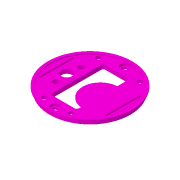
# Autodesk Inventor part: top_ring
Saved by Autodesk Inventor 2018 (Build 220112000, 112)
## iProperties
Created: 2019-01-25
Part Number: top_ring
Material: Generic
Document SubType Name: Modeling
Designer: Koki
Density: 1 g/cm^3
Appearance: Magenta
Author: Koki
Autodesk Inventor part; units mm, degrees
ref_plane "YZ Plane" through (0, 0, 0) normal (1, 0, 0) x (0, 1, 0)
ref_plane "XZ Plane" through (0, 0, 0) normal (0, 1, 0) x (-1, 0, 0)
ref_plane "XY Plane" through (0, 0, 0) normal (0, 0, 1) x (1, 0, 0)
ref_plane "Work Plane5" through (0, 4, 0) normal (0, 1, 0) x (1, 0, 0)
sketch "Sketch6" plane through (0, 4, 0) normal (0, 1, 0) x (1, 0, 0)
  circle A0 centre (0, 0) radius 38.1
  line L0 (15.875, -27.4963) -> (17.4625, -30.2459)
  line L1 (-15.875, -27.4963) -> (-17.4625, -30.2459)
  arc A1 (15.875, -27.4963) -> (27.4963, 15.875) centre (0, 0) ccw
  arc A2 (-27.4963, 15.875) -> (-15.875, -27.4963) centre (0, 0) ccw
  arc A3 (17.4625, -30.2459) -> (30.2459, 17.4625) centre (0, 0) ccw
  arc A4 (-30.2459, 17.4625) -> (-17.4625, -30.2459) centre (0, 0) ccw
  line L2 (0, 0) -> (-30.2459, 17.4625)
  line L3 (0, 0) -> (30.2459, 17.4625)
  line L4 (-15.875, 0) -> (19.5597, 0)
  dimension "d89" = 30
  dimension "d90" = 30
  constraints: 10 end point, 8 point on circle, 5 centre point, 3 coincident, 2 point on line, 1 horizontal
  measures "d89" angle of L4 L2
  measures "d90" angle of L4 L3
extrude "Extrusion6" add sketch "Sketch6" against normal blind 4 contours A0 | A1 L3 A3 L0 | L1 A4 L2 A2
sketch "Sketch7" plane through (0, 0, 0) normal (0, 0, 1) x (1, 0, 0)
  line L0 (0, 0) -> (0, 4)
  line L1 (-38.1, 4) -> (38.1, 4) projected
  line L2 (38.1, 4) -> (37.1, 4)
  line L3 (37.1, 4) -> (37.1, 5)
  line L4 (37.1, 5) -> (38.1, 5)
  line L5 (38.1, 5) -> (38.1, 4)
  line L6 (38.1, 4) -> (39.6875, 4)
  line L7 (39.6875, 4) -> (39.6875, 5)
  line L8 (39.6875, 5) -> (38.1, 5)
  line L9 (38.1, 5) -> (38.1, 4)
  dimension "d43" = 1
  dimension "d44" = 1
  dimension "d45" = 1.5875
  constraints: 18 end point, 4 parallel, 2 horizontal, 2 perpendicular, 1 point on line
  measures "d43" distance of L2.end L3.end
  measures "d44" distance of L3.end L4.end
  measures "d45" distance of L7.end L8.end
revolve "Revolution1" add sketch "Sketch7" angle 360 about axis through (0, 0, 0) along (0, 1, 0)
ref_plane "Work Plane3" through (0, 4, 0) normal (0, 1, 0) x (1, 0, 0)
sketch "Sketch10" plane through (0, 4, 0) normal (0, 1, 0) x (1, 0, 0)
  circle A0 centre (12.7, -30.48) radius 2.2
  line L0 (0, 0) -> (19.9404, 0)
  line L1 (0, 0) -> (0, -20.9357)
  circle A1 centre (12.7, 30.48) radius 2.2
  circle A2 centre (-12.7, -30.48) radius 2.2
  circle A3 centre (-12.7, 30.48) radius 2.2
  dimension "d46" = 30.48
  dimension "d47" = 12.7
  dimension "d48" = 4.4
  constraints: 4 centre point, 4 end point, 3 symmetric about line, 1 horizontal, 1 vertical, 3 other
  measures "d46" vertical distance of L0.start A0.centre
  measures "d47" horizontal distance of L0.start A0.centre
  measures "d48" diameter of A0
extrude "Extrusion7" cut sketch "Sketch10" against normal blind 4 contours A0 | A2
sketch "Sketch13" plane through (0, 4, 0) normal (0, 1, 0) x (1, 0, 0)
  line L0 (-32.258, -16.51) -> (-30.48, -16.51)
  line L1 (-30.48, -16.51) -> (-30.48, 16.51)
  line L2 (-30.48, 16.51) -> (-32.258, 16.51)
  line L3 (-32.258, 16.51) -> (-32.258, -16.51)
  point P0 (0, 0)
  dimension "d58" = 1.778
  dimension "d59" = 33.02
  dimension "d60" = 16.51
  dimension "d61" = 30.48
  constraints: 8 end point, 2 parallel, 1 horizontal, 1 perpendicular
  measures "d58" distance between parallel lines of L1 L3
  measures "d59" distance of L2.end L0.start
  measures "d60" distance from line of point (0, 0) L0
  measures "d61" distance from line of point (0, 0) L1
extrude "Extrusion10" cut sketch "Sketch13" along normal mid plane 3
mirror "Mirror1" about plane through (0, 0, 0) normal (1, 0, 0) of "Extrusion10"
chamfer "Chamfer2" distance 0.5 angle 45 4 edges at (-32.258, 4, 0) (-30.48, 4, 0) (32.258, 4, 0) (30.48, 4, 0)
sketch "Sketch14" plane through (0, 0, 0) normal (0, -1, 0) x (1, 0, 0)
  circle A0 centre (0, 33.02) radius 2.425
  point P0 (0, 0)
  dimension "d70" = 4.85
  dimension "d71" = 33.02
  constraints: 1 centre point
  measures "d70" diameter of A0
  measures "d71" distance of point (0, 0) A0.centre
extrude "Extrusion11" cut sketch "Sketch14" against normal blind 25.75
pattern_circular "Circular Pattern4" count 2 over 360 about axis through (0, 4.5, 0) along (0, -1, 0) of "Extrusion11"
sketch "Sketch15" plane through (0, 0, 0) normal (0, -1, 0) x (1, 0, 0)
  circle A0 centre (-12.7, 30.48) radius 2.2 projected
  circle A1 centre (-12.7, 30.48) radius 4
  line L0 (0, 0) -> (0, 13.7604)
  line L1 (0, 0) -> (23.7395, 0)
  circle A2 centre (12.7, 30.48) radius 4
  circle A3 centre (-12.7, -30.48) radius 2.2
  circle A4 centre (-12.7, -30.48) radius 4
  circle A5 centre (12.7, -30.48) radius 4
  dimension "d77" = 8
  constraints: 5 centre point, 4 end point, 4 symmetric about line, 2 coincident, 1 horizontal, 1 vertical, 4 other
  measures "d77" diameter of A1
extrude "Extrusion12" cut sketch "Sketch15" against normal blind 3 contours A1 | A2
sketch "Sketch16" plane through (0, 4, 0) normal (0, 1, 0) x (1, 0, 0)
  circle A0 centre (0, 33.02) radius 2.425 projected
  line L0 (0, 28.6899) -> (-3.75, 30.8549)
  line L1 (-3.75, 30.8549) -> (-3.75, 35.1851)
  line L2 (-3.75, 35.1851) -> (0, 37.3501)
  line L3 (0, 37.3501) -> (3.75, 35.1851)
  line L4 (3.75, 35.1851) -> (3.75, 30.8549)
  line L5 (3.75, 30.8549) -> (0, 28.6899)
  line L6 (0, 0) -> (11.6751, 0)
  circle A1 centre (0, -33.02) radius 2.425
  line L7 (0, -28.6899) -> (-3.75, -30.8549)
  line L8 (-3.75, -30.8549) -> (-3.75, -35.1851)
  line L9 (-3.75, -35.1851) -> (0, -37.3501)
  line L10 (0, -37.3501) -> (3.75, -35.1851)
  line L11 (3.75, -35.1851) -> (3.75, -30.8549)
  line L12 (3.75, -30.8549) -> (0, -28.6899)
  dimension "d80" = 7.5
  constraints: 26 end point, 8 symmetric about line, 2 coincident, 1 centre point, 1 horizontal, 14 other
  measures "d80" distance between parallel lines of L4 L1
extrude "Extrusion13" cut sketch "Sketch16" against normal blind 2.2
sketch "Sketch18" plane through (0, 4, 0) normal (0, 1, 0) x (1, 0, 0)
  circle A0 centre (19.558, 27.6098) radius 2.2
  line L0 (0, 0) -> (19.3787, 0)
  line L1 (0, 0) -> (0, 25.4098)
  circle A1 centre (-19.558, 27.6098) radius 2.2
  dimension "d83" = 4.4
  dimension "d84" = 27.6098
  dimension "d85" = 19.558
  constraints: 4 end point, 2 centre point, 1 horizontal, 1 symmetric about line, 1 vertical, 1 other
  measures "d83" diameter of A0
  measures "d84" vertical distance of L0.start A0.centre
  measures "d85" horizontal distance of L0.start A0.centre
extrude "Extrusion14" cut sketch "Sketch18" against normal blind 10
sketch "Sketch20" plane through (0, 0, 0) normal (0, 1, 0) x (-1, 0, 0)
  line L0 (12.5, 25) -> (-12.5, 25)
  line L1 (-12.5, 25) -> (-12.5, -25)
  line L2 (-12.5, -25) -> (12.5, -25)
  line L3 (12.5, -25) -> (12.5, 25)
  point P0 (0, 0)
  dimension "d94" = 50
  dimension "d95" = 25
  dimension "d96" = 25
  dimension "d97" = 12.5
  constraints: 8 end point, 2 parallel, 1 horizontal, 1 perpendicular
  measures "d94" distance of L0.end L1.end
  measures "d95" distance of L0.start L0.end
  measures "d96" distance from line of point (0, 0) L0
  measures "d97" distance from line of point (0, 0) L1
extrude "Extrusion15" cut sketch "Sketch20" along normal blind 10
fillet "Fillet5" radius 2 4 edges at (12.5, 2, 25) (-12.5, 2, 25) (-12.5, 2, -25) (12.5, 2, -25)
sketch "Sketch21" plane through (0, 0, 0) normal (0, -1, 0) x (1, 0, 0)
  circle A0 centre (-19.558, -27.6098) radius 2.2 projected
  circle A1 centre (-19.558, -27.6098) radius 4
  circle A2 centre (19.558, -27.6098) radius 2.2 projected
  circle A3 centre (19.558, -27.6098) radius 4
  circle A4 centre (-12.7, 30.48) radius 4 projected
  point P0 (0, 0)
  dimension "d102" = 8
  dimension "d103" = 8
  constraints: 2 centre point, 2 coincident
  measures "d102" diameter of A1
  measures "d103" diameter of A3
extrude "Extrusion16" cut sketch "Sketch21" against normal blind 3 contours A1 | A3
sketch "Sketch22" plane through (0, 4, 0) normal (0, 1, 0) x (1, 0, 0)
  circle A0 centre (22, 0) radius 5
  line L0 (0, 0) -> (0, -19.8965)
  circle A1 centre (-22, 0) radius 5
  circle A2 centre (20, 12) radius 2.75
  line L1 (0, 0) -> (8.5328, 0)
  circle A3 centre (20, -12) radius 2.75
  circle A4 centre (-20, 12) radius 2.75
  circle A5 centre (-20, -12) radius 2.75
  dimension "d106" = 10
  dimension "d107" = 22
  dimension "d110" = 5.5
  dimension "d111" = 20
  dimension "d112" = 12
  constraints: 6 centre point, 4 end point, 4 symmetric about line, 1 horizontal, 1 vertical, 4 other
  measures "d106" diameter of A0
  measures "d107" distance of L0.start A0.centre
  measures "d110" diameter of A2
  measures "d111" horizontal distance of L0.start A2.centre
  measures "d112" vertical distance of L0.start A2.centre
extrude "Extrusion17" cut sketch "Sketch22" against normal blind 5 contours A1 | A4 | A5
sketch "Sketch23" plane through (0, 0, 0) normal (0, -1, 0) x (1, 0, 0)
  circle A0 centre (9.736, 0) radius 16.715
  point P0 (0, 0)
  dimension "d114" = 33.43
  dimension "d121" = 0
  dimension "d122" = 9.736
  constraints: 1 centre point
  measures "d114" diameter of A0
  measures "d121" vertical distance of point (0, 0) A0.centre
  measures "d122" distance of point (0, 0) A0.centre
extrude "Extrusion18" add sketch "Sketch23" along normal blind 0.5 and the other way blind 0.5
sketch "Sketch24" plane through (9.736, -0.5, 0) normal (0, -1, 0) x (1, 0, 0)
  arc A0 (2.764, 16.4849) -> (2.764, -16.4849) centre (0, 0) ccw projected
  circle A1 centre (0, 0) radius 12
  point P0 (-9.736, 0)
  point P1 (2.5, 18.3303)
  point P2 (2.5, -18.3303)
  point P3 (2.764, 18.2924)
  point P4 (2.764, -18.2924)
  point P5 (-4.49, 25)
  point P6 (-22.236, 12.2768)
  dimension "d117" = 24
  constraints: 1 centre point, 1 coincident, 1 other
  measures "d117" diameter of A1
extrude "Extrusion19" add sketch "Sketch24" along normal blind 2
fillet "Fillet7" radius 2 1 edges at (12.5, 0.5, 0)
fillet "Fillet8" radius 2 2 edges at (22.4951, 0, 10.7979) (22.4951, 0, -10.7979)
equation "\"d60\" = 0.5 * d59"
equation "\"d96\" = 0.5 * d94"
equation "\"d97\" = 0.5 * d95"
equation "\"d103\" = d102"
body "Solid1"
